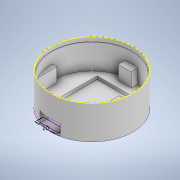
# Autodesk Inventor part: t1
Saved by Autodesk Inventor 2022.2 (Build 262287000, 287)
## iProperties
Created: 2022-04-05
Part Number: t1
Material: Generic
Document SubType Name: Modeling
Designer: 21towe
Density: 1 g/cm^3
Appearance: Default
Author: 21towe
Autodesk Inventor part; units mm, degrees
ref_plane "YZ Plane" through (0, 0, 0) normal (1, 0, 0) x (0, 1, 0)
ref_plane "XZ Plane" through (0, 0, 0) normal (0, 1, 0) x (-1, 0, 0)
ref_plane "XY Plane" through (0, 0, 0) normal (0, 0, 1) x (1, 0, 0)
sketch "Sketch1" plane through (0, 0, 0) normal (0, 1, 0) x (-1, 0, 0)
  circle A0 centre (0, 0) radius 18.75
  circle A1 centre (0, 0) radius 19.25
  dimension "d0" = 37.5
  dimension "d1" = 38.5
  constraints: 2 centre point, 2 coincident
  measures "d0" diameter of A0
  measures "d1" diameter of A1
extrude "Extrusion1" add sketch "Sketch1" along normal blind 0.5 contours A0 | A1
sketch "Sketch2" plane through (0, 0.5, 0) normal (0, 1, 0) x (1, 0, 0)
  line L0 (-10, -12.5) -> (8.5, -12.5)
  line L1 (10, -11) -> (10, 12.5)
  line L2 (10, 12.5) -> (-10, 12.5)
  line L3 (-10, 12.5) -> (-10, -12.5)
  line L4 (-10, -12.5) -> (10, 12.5) construction
  line L5 (10, -12.5) -> (-10, 12.5) construction
  line L6 (8.5, -12.5) -> (8.5, -14)
  line L7 (8.5, -14) -> (11.5, -14)
  line L8 (11.5, -14) -> (11.5, -11)
  line L9 (11.5, -11) -> (8.5, -14) construction
  line L10 (8.5, -11) -> (11.5, -14) construction
  line L11 (11.5, -11) -> (10, -11)
  line L12 (8.8, -11) -> (8.5, -11)
  circle A0 centre (0, 0) radius 19.25
  dimension "d4" = 20
  dimension "d5" = 25
  dimension "d6" = 3
  dimension "d7" = 3
  constraints: 26 end point, 5 parallel, 4 midpoint, 3 horizontal, 3 perpendicular, 1 centre point, 1 coincident, 1 point on line
  measures "d4" distance of L2.end L1.end
  measures "d5" distance of L1.end L5.start
  measures "d6" distance of L7.end L6.end
  measures "d7" distance of L6.end L10.start
extrude "Extrusion2" add sketch "Sketch2" along normal blind 3.25
sketch "Sketch3" plane through (0, 3.75, 0) normal (0, 1, 0) x (1, 0, 0)
  circle A0 centre (0, 0) radius 19.25
  circle A1 centre (0, 0) radius 19.25 projected
  line L0 (0, 16.25) -> (-3, 16.25)
  line L1 (-3, 16.25) -> (-3, 18.2551)
  line L2 (0, 16.25) -> (3, 16.25)
  line L3 (3, 16.25) -> (3, 18.2551)
  circle A2 centre (0, 0) radius 19.25 projected
  line L4 (18.5, 0) -> (12.5, 0)
  line L5 (12.5, 0) -> (12.5, 2.75)
  line L6 (12.5, 2.75) -> (12.5, -2.75)
  line L7 (12.5, -2.75) -> (10, -2.75)
  line L8 (10, 12.5) -> (10, -11) projected
  line L9 (10, -2.75) -> (10, 2.75)
  line L10 (10, 2.75) -> (12.5, 2.75)
  line L11 (-6, -17.5) -> (-6, -12.5)
  line L12 (8.5, -12.5) -> (-10, -12.5) projected
  line L13 (-6, -12.5) -> (-13.6382, -12.5)
  line L14 (-18.5, 0) -> (-16.5, 0)
  line L15 (-16.5, 0) -> (-16.5, -8.3666)
  line L16 (3, 18.2551) -> (3, 15.4901)
  line L17 (3, 15.4901) -> (-3, 15.4901)
  line L18 (-3, 15.4901) -> (-3, 16.25)
  circle A3 centre (0, 0) radius 18.75
  line L19 (-3, 18.2551) -> (-3, 18.5084)
  line L20 (3, 18.2551) -> (3, 18.5084)
  line L21 (-18.5, 0) -> (-18.75, 0)
  line L22 (-16.5, -8.3666) -> (-16.5, -8.9058)
  line L23 (-6, -17.5) -> (-6, -17.7641)
  line L24 (-13.6382, -12.5) -> (-13.9754, -12.5)
  dimension "d20" = 6
  dimension "d21" = 2.75
  dimension "d22" = 5.5
  dimension "d23" = 2
  dimension "d24" = 2.765
  dimension "d25" = 37.5
  constraints: 46 end point, 9 perpendicular, 7 point on line, 6 point on circle, 4 vertical, 2 centre point, 1 coincident, 1 horizontal, 1 parallel, 1 other
  measures "d20" distance of L4.start L4.end
  measures "d21" distance of L4.end L5.end
  measures "d22" distance of L5.end L6.end
  measures "d23" distance of L14.start L14.end
  measures "d24" distance of L3.end L16.end
  measures "d25" diameter of A3
extrude "Extrusion3" cut sketch "Sketch3" against normal blind 1.75 contours L18 L17 L16 L3 L20 A3 L23 L11 L12 L13 L24 L22 L15 L14 L21 L19 L1
extrude "Extrusion4" add sketch "Sketch3" along normal blind 5 contours A0 | L2 L16 L17 L18 L0 | L0 L1 L19 A3 L20 L3 L2 | L21 L14 L15 L22 A3 | A3 L24 L13 L12 L11 L23 | L6 L7 L8 L10 L5
sketch "Sketch4" plane through (0, 8.75, 0) normal (0, 1, 0) x (1, 0, 0)
  circle A0 centre (0, 0) radius 19.25
  circle A1 centre (0, 0) radius 18.75
  constraints: 2 centre point, 2 coincident
extrude "Extrusion5" add sketch "Sketch4" along normal blind 5
sketch "Sketch5" plane through (0, 13.75, 0) normal (0, 1, 0) x (1, 0, 0)
  circle A0 centre (0, 0) radius 19
  circle A1 centre (0, 0) radius 19.25
  dimension "d32" = 38
  constraints: 2 centre point, 2 coincident
  measures "d32" diameter of A0
extrude "Extrusion6" add sketch "Sketch5" along normal blind 2
sketch "Sketch6" plane through (0, 15.75, 0) normal (0, 1, 0) x (1, 0, 0)
  circle A0 centre (0, 0) radius 19.25 projected
  circle A1 centre (0, 0) radius 19 projected
  line L0 (0, -19.25) -> (-0.1562, -19.25)
  line L1 (-0.1562, -19.25) -> (-0.1562, -18.8969)
  line L2 (-0.1562, -18.8969) -> (0, -18.8969)
  line L3 (0, -18.8969) -> (0, -19.25)
  point P0 (0, -19)
  point P1 (-0.1562, -18.9994)
  point P2 (-0.1562, -19.2494)
  constraints: 8 end point, 2 parallel, 1 horizontal, 1 perpendicular, 2 other
extrude "Extrusion7" add sketch "Sketch6" along normal blind 1 contours L1 A1 L3 A0 picked at (-0.1388, -19.083)
sketch "Sketch7" plane through (0, 15.75, 19.25) normal (1, 0, 0) x (0, 0, -1)
  line L0 (0.25, 0) -> (0, 0) projected
  line L1 (0, 0) -> (0.125, 0)
  circle A0 centre (0.125, 0) radius 0.125
  line L2 (0.125, 0) -> (0.25, 0)
  point P0 (19.25, -15.75)
  dimension "d37" = 0.125
  constraints: 4 end point, 1 coincident, 1 horizontal, 1 midpoint, 3 other
  measures "d37" distance of L0.end L1.end
extrude "Extrusion8" cut sketch "Sketch6" along normal blind 1 contours L1 A1 L3 A0 | L1 L2 L3 A1 picked at (-0.1388, -19.083) picked at (-0.0868, -18.9312)
sketch3d "3D Sketch1"
  arc A0 (0, 15.75, 19) -> (-19, 15.75, 0) centre (0, 15.75, 0) ccw
  arc A1 (-19, 15.75, 0) -> (0, 15.75, -19) centre (0, 15.75, 0) ccw
  arc A2 (0, 15.75, -19) -> (19, 15.75, 0) centre (0, 15.75, 0) ccw
  arc A3 (19, 15.75, 0) -> (0, 15.75, 19) centre (0, 15.75, 0) ccw
sweep "Sweep1" add profiles "Sketch7" path "3D Sketch1" picked at (0.0448, 0.0159) contours L0 A0
sketch "Sketch8" plane through (0, 2, 0) normal (0, 1, 0) x (1, 0, 0)
  line L0 (-6, -17.7641) -> (-6, -12.5) projected
  line L1 (-6, -16.8786) -> (4, -16.8786)
  line L2 (4, -16.8786) -> (4, -19.7767)
  line L3 (4, -19.7767) -> (-6, -19.7767)
  line L4 (-6, -19.7767) -> (-6, -16.8786)
  point P0 (0, 0)
  dimension "d42" = 10
  constraints: 8 end point, 2 parallel, 1 horizontal, 1 perpendicular, 1 point on line
  measures "d42" distance of L2.end L3.end
extrude "Extrusion9" cut sketch "Sketch8" against normal blind 1.75
extrude "Extrusion10" cut sketch "Sketch8" along normal blind 3.25
sketch "Sketch9" plane through (-6, 2, 12.5) normal (1, 0, 0) x (0, 0, -1)
  point P0 (12.5, -2)
sketch "Sketch10" plane through (0, 2, 0) normal (0, 1, 0) x (1, 0, 0)
  line L0 (-6, -16.8786) -> (4, -16.8786) projected
  line L1 (-6, -12.5) -> (8.5, -12.5) projected
  line L2 (-6, -16.8786) -> (4.0086, -16.8786)
  line L3 (4.0086, -16.8786) -> (4.0086, -12.5)
  line L4 (4.0086, -12.5) -> (-6, -12.5)
  line L5 (-6, -12.5) -> (-6, -16.8786)
  point P0 (0, 0)
  constraints: 8 end point, 2 parallel, 1 horizontal, 1 perpendicular, 1 point on line
extrude "Extrusion11" cut sketch "Sketch10" against normal blind 1.75
body "Solid1"
